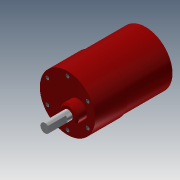
# Autodesk Inventor part: DC_motor_with_encoder
Saved by Autodesk Inventor 2015 (Build 190159000, 159)
## iProperties
Created: 2013-11-16
Part Number: DC_motor_with_encoder
Material: Generic
Document SubType Name: Modeling
Designer: idle-rug
Density: 1 g/cm^3
Appearance: Default
Author: idle-rug
Autodesk Inventor part; units mm, degrees
ref_plane "YZ Plane" through (0, 0, 0) normal (1, 0, 0) x (0, 1, 0)
ref_plane "XZ Plane" through (0, 0, 0) normal (0, 1, 0) x (-1, 0, 0)
ref_plane "XY Plane" through (0, 0, 0) normal (0, 0, 1) x (1, 0, 0)
sketch "Sketch1" plane through (0, 0, 0) normal (0, 1, 0) x (-1, 0, 0)
  circle A0 centre (0, 0) radius 18.4
  dimension "d0" = 36.8
  constraints: 1 centre point, 1 coincident
  measures "d0" diameter of A0
extrude "Extrusion1" add sketch "Sketch1" along normal blind 22
sketch "Sketch2" plane through (0, 22, 0) normal (0, 1, 0) x (1, 0, 0)
  circle A0 centre (0, 0) radius 18.4 projected
  circle A1 centre (0, 0) radius 17.9
  dimension "d3" = 35.8
  constraints: 1 centre point, 1 coincident
  measures "d3" diameter of A1
extrude "Extrusion2" add sketch "Sketch2" along normal blind 30 contours A1
fillet "Fillet1" radius 0.5 1 edges at (18.4, 22, 0)
sketch "Sketch3" plane through (0, 0, 0) normal (0, -1, 0) x (1, 0, 0)
  circle A0 centre (0, 0) radius 18.4 projected
  line L0 (0, 0) -> (7, 0)
  circle A1 centre (7, 0) radius 6
  dimension "d7" = 7
  dimension "d8" = 12
  constraints: 2 end point, 1 centre point, 1 coincident, 1 horizontal
  measures "d7" distance of L0.start L0.end
  measures "d8" diameter of A1
extrude "Extrusion3" add sketch "Sketch3" along normal blind 6.5 contours A1
sketch "Sketch4" plane through (7, -6.5, 0) normal (0, -1, 0) x (1, 0, 0)
  circle A0 centre (0, 0) radius 6 projected
  circle A1 centre (0, 0) radius 3
  point P0 (-7, 0)
  dimension "d11" = 6
  constraints: 1 centre point, 1 coincident
  measures "d11" diameter of A1
extrude "Extrusion4" add sketch "Sketch4" along normal blind 3.5 contours A1
sketch "Sketch5" plane through (7, -10, 0) normal (0, -1, 0) x (1, 0, 0)
  circle A0 centre (0, 0) radius 3 projected
  point P0 (-7, 0)
extrude "Extrusion5" add sketch "Sketch5" along normal blind 12
chamfer "Chamfer1" distance 1 angle 45 1 edges at (1, -6.5, 0)
sketch "Sketch6" plane through (7, -22, 0) normal (0, -1, 0) x (1, 0, 0)
  circle A0 centre (0, 0) radius 3 projected
  line L0 (3, 0) -> (2.4, 0)
  line L1 (3.4, -3) -> (2, -3)
  line L2 (2, -3) -> (2, 3)
  line L3 (2, 3) -> (3.4, 3)
  line L4 (3.4, 3) -> (3.4, -3)
  line L5 (3.4, -3) -> (2, 3) construction
  line L6 (2, -3) -> (3.4, 3) construction
  point P0 (-7, 0)
  point P1 (2.7, 0)
  dimension "d19" = 0.6
  constraints: 14 end point, 3 midpoint, 2 horizontal, 2 parallel, 1 horizontal alignment, 1 perpendicular, 1 other
  measures "d19" distance of L0.start L0.end
extrude "Extrusion6" cut sketch "Sketch6" against normal blind 12 contours A0 L2 | A0 L2 L3 L4 L1 picked at (2.1409, -0.5898)
sketch "Sketch7" plane through (0, 0, 0) normal (0, -1, 0) x (1, 0, 0)
  circle A0 centre (0, 0) radius 18.4 projected
  circle A1 centre (0, 0) radius 15.5
  circle A2 centre (0, 15.5) radius 1.2
  circle A3 centre (0, -15.5) radius 1.2
  circle A4 centre (-13.4234, -7.75) radius 1.2
  circle A5 centre (13.4234, -7.75) radius 1.2
  circle A6 centre (-13.4234, 7.75) radius 1.2
  circle A7 centre (13.4234, 7.75) radius 1.2
  dimension "d22" = 31
  dimension "d23" = 2.4
  dimension "d24" = 2.4
  dimension "d28" = 2.4
  dimension "d29" = 2.4
  dimension "d32" = 2.4
  dimension "d33" = 15.5
  dimension "d34" = 2.4
  constraints: 7 centre point, 5 point on circle, 1 coincident
  measures "d22" diameter of A1
  measures "d23" diameter of A2
  measures "d24" diameter of A3
  measures "d28" diameter of A4
  measures "d29" diameter of A5
  measures "d32" diameter of A6
  measures "d33" distance of A4.centre A6.centre
  measures "d34" diameter of A7
hole "Hole1" at (13.4234, 0, 7.75) at (13.4234, 0, -7.75) at (0, 0, 15.5) at (-13.4234, 0, 7.75) at (-13.4234, 0, -7.75) at (0, 0, -15.5) direction (0, 1, 0) diameter 2.459 depth 3 thread size "M3x0.5" designation "M3" class "6H" standard "GB Metric profile"
body "Solid1"
